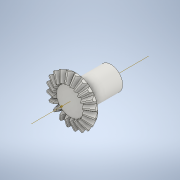
# Autodesk Inventor part: Kegelrad2
Saved by Autodesk Inventor 2021 (Build 250183000, 183)
## iProperties
CustomPartVersion: 1
Created: 2021-01-23
Part Number: Kegelrad2
Material: Steel, Mild
Document SubType Name: Blech
Designer: LETPJG
Categories: <?xml version="1.0" encoding="UTF-16"?> <MemberInstance><Categories><FamilyTemplate><FamilyTemplateParameter ValueType="xs:double" Id="1" ObjectReferenceKey="da_z" ObjectType="kUserParameterObject"/><FamilyTemplateParameter ValueType="xs:double" Id="2" ObjectReferenceKey="da_b" ObjectType="kUserParameterObject"/><FamilyTemplateParameter ValueType="xs:double" Id="3" ObjectReferenceKey="da_beta" ObjectType="kUserParameterObject"/><FamilyTemplateParameter ValueType="xs:double" Id="4" ObjectReferenceKey="da_dae" ObjectType="kUserParameterObject"/><FamilyTemplateParameter ValueType="xs:double" Id="5" ObjectReferenceKey="da_ve" ObjectType="kUserParameterObject"/><FamilyTemplateParameter ValueType="xs:double" Id="6" ObjectReferenceKey="da_omega" ObjectType="kUserParameterObject"/><FamilyTemplateParameter ValueType="xs:string" Id="7" ObjectReferenceKey="EAIAABAAAAAAHwAAAAAAAIAAAAAAAAAA" ObjectType="83914240" SubObjectId="SurfaceGeometry"/></FamilyTemplate><ParamToTemplateMap><ParamToTemplate CategoryParameter="//CategoryParameter[@InternalName='046C89C9-8512-4d59-83FE-43B91F4F132A']" TemplateParameter="1"/><ParamToTemplate CategoryParameter="//CategoryParameter[@InternalName='2552DF32-E462-4b46-AEBF-C6C7768E72AC']" TemplateParameter="2"/><ParamToTemplate CategoryParameter="//CategoryParameter[@InternalName='C9EE641D-15FC-4fae-A226-E94C4372FDD7']" TemplateParameter="3"/><ParamToTemplate><ParamToTemplate CategoryParameter="//CategoryParameter[@InternalName='00B6519A-459B-49c7-AD84-2E56D39A5744']" ConstantValue="-0.000000"/></ParamToTemplate><ParamToTemplate><ParamToTemplate CategoryParameter="//CategoryParameter[@InternalName='04B31F0E-C7A6-4894-AA32-9629BEFACF47']" ConstantValue="1.000000"/></ParamToTemplate><ParamToTemplate><ParamToTemplate CategoryParameter="//CategoryParameter[@InternalName='43CBEC2E-7847-49e7-A936-2F7889FCB2D9']" ConstantValue="0.200000"/></ParamToTemplate><ParamToTemplate><ParamToTemplate CategoryParameter="//CategoryParameter[@InternalName='B1EFC894-105D-4ebd-86BF-FA20ED196853']" ConstantValue="0.300000"/></ParamToTemplate><ParamToTemplate><ParamToTemplate CategoryParameter="//CategoryParameter[@InternalName='51175063-3D10-4879-93E8-6246FE8B403D']" ConstantValue="2060000000.000000"/></ParamToTemplate><ParamToTemplate><ParamToTemplate CategoryParameter="//CategoryParameter[@InternalName='A3A52E27-4454-46a9-B0BD-C932399B70AF']" ConstantValue="0.300000"/></ParamToTemplate><ParamToTemplate CategoryParameter="//CategoryParameter[@InternalName='2A200944-5A8C-41ca-B96E-8520D2E510F1']" TemplateParameter="4"/><ParamToTemplate><ParamToTemplate CategoryParameter="//CategoryParameter[@InternalName='1A637F62-92C8-44bc-B81F-10802510B579']" ConstantValue="1.285835"/></ParamToTemplate><ParamToTemplate CategoryParameter="//CategoryParameter[@InternalName='B52DD4BE-6863-48fb-BF58-89EF6F9EC65C']" TemplateParameter="5"/><ParamToTemplate><ParamToTemplate CategoryParameter="//CategoryParameter[@InternalName='3956BFF2-84D2-457d-93C2-9B0613DEBA67']" ConstantValue="0.252655"/></ParamToTemplate><ParamToTemplate CategoryParameter="//CategoryParameter[@InternalName='739CFA02-461B-4bf8-8049-181FCAD8B28F']" TemplateParameter="6"/><ParamToTemplate><ParamToTemplate CategoryParameter="//CategoryParameter[@InternalName='A27E999F-E2CE-4481-8A2A-EBF499C4C3C5']" ConstantValue="-0.000000"/></ParamToTemplate><ParamToTemplate><ParamToTemplate CategoryParameter="//CategoryParameter[@InternalName='9E1B4470-B2D3-4ff1-B813-535BB4CDF51A']" ConstantValue="3520000.000000"/></ParamToTemplate><ParamToTemplate><ParamToTemplate CategoryParameter="//CategoryParameter[@InternalName='F8452263-BFF6-458c-9FB1-07C4B99E95CD']" ConstantValue="11400000.000000"/></ParamToTemplate><ParamToTemplate><ParamToTemplate CategoryParameter="//CategoryParameter[@InternalName='3E3BB259-FD49-497f-8171-6EBC954A3479']" ConstantValue="2.000000"/></ParamToTemplate><ParamToTemplate CategoryParameter="//CategoryParameter[@InternalName='27C3BAF2-7550-4e4b-AE2C-0DB134B7D9B7']" TemplateParameter="7"/></ParamToTemplateMap><Category DisplayName="Gear" InternalName="DC85795E-93AB-48d5-8EEE-5A27447B64BD" Mnemonic="Gear"><CategoryParameter DisplayName="z" InternalName="046C89C9-8512-4d59-83FE-43B91F4F132A" Mnemonic="z"/><CategoryParameter DisplayName="b" InternalName="2552DF32-E462-4b46-AEBF-C6C7768E72AC" Mnemonic="b"/><CategoryParameter DisplayName="||b|" InternalName="C9EE641D-15FC-4fae-A226-E94C4372FDD7" Mnemonic="beta"/><CategoryParameter DisplayName="x" InternalName="00B6519A-459B-49c7-AD84-2E56D39A5744" Mnemonic="x"/><CategoryParameter DisplayName="a*" InternalName="04B31F0E-C7A6-4894-AA32-9629BEFACF47" Mnemonic="a"/><CategoryParameter DisplayName="c*" InternalName="43CBEC2E-7847-49e7-A936-2F7889FCB2D9" Mnemonic="c"/><CategoryParameter DisplayName="r|.f|*" InternalName="B1EFC894-105D-4ebd-86BF-FA20ED196853" Mnemonic="rf"/><CategoryParameter DisplayName="E" InternalName="51175063-3D10-4879-93E8-6246FE8B403D" Mnemonic="E"/><CategoryParameter DisplayName="||m|" InternalName="A3A52E27-4454-46a9-B0BD-C932399B70AF" Mnemonic="mi"/><Category DisplayName="BevelGear" InternalName="0C98F69A-0C2B-4791-B2FE-7691BB227E77" Mnemonic="BevelGear"><CategoryParameter DisplayName="d|.ae|" InternalName="2A200944-5A8C-41ca-B96E-8520D2E510F1" Mnemonic="dae"/><CategoryParameter DisplayName="d|.ai|" InternalName="1A637F62-92C8-44bc-B81F-10802510B579" Mnemonic="dai"/><CategoryParameter DisplayName="A|.e|" InternalName="B52DD4BE-6863-48fb-BF58-89EF6F9EC65C" Mnemonic="ve"/><CategoryParameter DisplayName="A|.i|" InternalName="3956BFF2-84D2-457d-93C2-9B0613DEBA67" Mnemonic="vi"/><CategoryParameter DisplayName="||S|" InternalName="739CFA02-461B-4bf8-8049-181FCAD8B28F" Mnemonic="omega"/><CategoryParameter DisplayName="x|.t|" InternalName="A27E999F-E2CE-4481-8A2A-EBF499C4C3C5" Mnemonic="xt"/><CategoryParameter DisplayName="||s||.Flim|" InternalName="9E1B4470-B2D3-4ff1-B813-535BB4CDF51A" Mnemonic="sFlim"/><CategoryParameter DisplayName="||s||.Hlim|" InternalName="F8452263-BFF6-458c-9FB1-07C4B99E95CD" Mnemonic="sHlim"/><CategoryParameter DisplayName="Typ" InternalName="3E3BB259-FD49-497f-8171-6EBC954A3479" Mnemonic="type"/><CategoryParameter DisplayName="PitchDiameter" InternalName="27C3BAF2-7550-4e4b-AE2C-0DB134B7D9B7" Mnemonic="IDS_PITCHDIAM"/></Category></Category></Categories></MemberInstance>
Mass: 60.9118 g
Surface Area: 34.3074 cm^2
Volume: 7.7496 cm^3
Density: 7.86 g/cm^3
Appearance: Steel
Sheet Metal Rule: Standard
Author: LETPJG
Autodesk Inventor part; units mm, degrees
ref_plane "Netzebene2" through (0, 0, 0) normal (0.9876883, 0.1564345, 0) x (0, 0, 1)
sketch "Skizze des Zahnradkörpers" plane through (0, 0, 0) normal (1, 0, 0) x (0, 1, 0)
  line L0 (0, 0) -> (9.463344, -6.073313) construction
  line L1 (9.463344, -6.073313) -> (10.447214, -4.105573)
  line L2 (10.447214, -4.105573) -> (0, 0) construction
  line L3 (10, -5) -> (0, 0) construction
  line L4 (5.823707, -3.737494) -> (6.429177, -2.526554)
  line L5 (9.463344, -6.073313) -> (5.823707, -3.737494)
  line L6 (10.447214, -4.105573) -> (6.429177, -2.526554)
  line L7 (0, -39.386751) -> (0, 6.564458)
  line L8 (0, -5) -> (10.447214, -5) construction
  dimension "d0" = 20
  dimension "d1" = 18.92669
  dimension "d2" = 20.89443
  dimension "d3" = 4.3
  dimension "d4" = 4.10557
  constraints: 16 end point, 4 point on line, 3 perpendicular, 2 collinear, 1 horizontal alignment, 1 vertical alignment
  measures "d0" diameter of L3.start L7
  measures "d1" diameter of L0.end L7
  measures "d2" diameter of L1.end L7
  measures "d3" distance between parallel lines of L1 L4
  measures "d4" vertical distance of L1.end L0.start
revolve "Zahnradkörper" add sketch "Skizze des Zahnradkörpers" angle 360 about axis through (0, 0, 0) along (0, 0, 1)
ref_plane "Zahnebene" through (0, 10, -5) normal (0, -0.8944272, 0.4472136) x (1, 0, 0)
sketch "Startskizze" plane through (0, 10, -5) normal (0, -0.8944272, 0.4472136) x (1, 0, 0)
  line L0 (0, -23.505131) -> (0, 10.644758)
  arc A0 (-0.366347, -1.464) -> (-1.669997, 1.601878) centre (-8.211235, -2.989641) ccw
  arc A1 (1.669997, 1.601878) -> (0.366347, -1.464) centre (8.211235, -2.989641) ccw
  line L1 (-0.366347, -1.464) -> (0.366347, -1.464)
  arc A2 (1.669997, 1.601878) -> (-1.669997, 1.601878) centre (0, -22.36068) ccw
  dimension "d7" = 7.99186
  dimension "d8" = 8.21124
  dimension "d9" = 19.37104
  dimension "d57" = 24.02068
  dimension "d58" = 20.89668
  constraints: 6 point on circle, 3 centre point, 3 symmetric about line, 2 end point, 1 coincident, 1 perpendicular, 1 other
  measures "d7" radius of A0
  measures "d8" horizontal distance of point (0, -22.361) A0.centre
  measures "d9" vertical distance of point (0, -22.361) A0.centre
  measures "d57" radius of A2
  measures "d58" distance from line of A2.centre L1
ref_plane "Endebene" through (0, 6.055576, -3.027788) normal (0, -0.8944272, 0.4472136) x (1, 0, 0)
sketch "Endskizze" plane through (0, 6.055576, -3.027788) normal (0, -0.8944272, 0.4472136) x (1, 0, 0)
  line L0 (0, -15.35404) -> (0, 6.953444)
  arc A0 (-0.221844, -0.886536) -> (-1.011279, 0.970029) centre (-4.972376, -1.8104) ccw
  arc A1 (1.011279, 0.970029) -> (0.221844, -0.886536) centre (4.972376, -1.8104) ccw
  line L1 (-0.221844, -0.886536) -> (0.221844, -0.886536)
  arc A2 (1.011279, 0.970029) -> (-1.011279, 0.970029) centre (0, -13.54068) ccw
  dimension "d12" = 4.83953
  dimension "d15" = 4.97238
  dimension "d16" = 11.73028
  dimension "d59" = 14.54591
  dimension "d60" = 12.65414
  constraints: 6 point on circle, 3 centre point, 3 symmetric about line, 2 end point, 1 coincident, 1 other
  measures "d12" radius of A0
  measures "d15" horizontal distance of A0.centre point (0, -13.541)
  measures "d16" vertical distance of A0.centre point (0, -13.541)
  measures "d59" radius of A2
  measures "d60" distance from line of A2.centre L1
loft "Loft" cut profiles "Startskizze", "Endskizze"
pattern_circular "Circular Pattern" count 20 over 360 about axis through (0, 0, 0) along (0, 0, 1) of "Loft"
sketch3d "3D-Skizze rechts"
ref_plane "Endebene rechts" through (-1.195497, 5.936395, -3.027788) normal (0.1765786, -0.8768238, 0.4472136) x (0.9803188, 0.1974209, 0)
sketch "Endskizze rechts" plane through (-1.195497, 5.936395, -3.027788) normal (0.1765786, -0.8768238, 0.4472136) x (0.9803188, 0.1974209, 0)
  arc A0 (-0.221844, -0.886536) -> (-1.011279, 0.970029) centre (-4.972376, -1.8104) ccw
  line L0 (0, -18.59884) -> (0, 8.824815)
  arc A1 (1.011279, 0.970029) -> (0.221844, -0.886536) centre (4.972376, -1.8104) ccw
  line L1 (-0.221844, -0.886536) -> (0.221844, -0.886536)
  arc A2 (1.011279, 0.970029) -> (-1.011279, 0.970029) centre (0, -13.54068) ccw
  dimension "d70" = 4.97238
  dimension "d71" = 11.73028
  dimension "d72" = 4.83953
  dimension "d73" = 12.65414
  dimension "d74" = 14.54591
  constraints: 6 point on circle, 3 centre point, 3 symmetric about line, 2 end point, 1 coincident, 1 perpendicular, 1 other
  measures "d70" horizontal distance of A2.centre A0.centre
  measures "d71" vertical distance of point (0, -13.541) A0.centre
  measures "d72" radius of A0
  measures "d73" distance from line of point (0, -13.541) L1
  measures "d74" radius of A2
feature "Erhebung rechts" [suppressed]
pattern_circular "Runde Anordnung rechts" [suppressed]
sketch3d "3D-Skizze links"
ref_plane "Endebene links" through (1.238266, 5.936395, -3.054356) normal (-0.1823679, -0.8742937, 0.449836) x (0.9789304, -0.204194, 0)
sketch "Endskizze links" plane through (1.238266, 5.936395, -3.054356) normal (-0.1823679, -0.8742937, 0.449836) x (0.9789304, -0.204194, 0)
  line L0 (0, -29.014384) -> (0, 11.991661)
  arc A0 (-0.221844, -0.866613) -> (-1.011279, 0.989952) centre (-4.972376, -1.790477) ccw
  arc A1 (1.011279, 0.989952) -> (0.221844, -0.866613) centre (4.972376, -1.790477) ccw
  line L1 (-0.221844, -0.866613) -> (0.221844, -0.866613)
  ellipse E0 centre (0, -2.256494) end of major axis (6.429177, -2.256494) minor radius 2.892075
  arc A2 (1.011279, 0.989952) -> (-1.011279, 0.989952) centre (0, -13.520757) ccw
  dimension "d56" = 2.89207
  dimension "d30" = 4.83953
  dimension "d31" = 4.97238
  dimension "d32" = 11.73028
  dimension "d61" = 14.54591
  dimension "d62" = 12.65414
  constraints: 6 point on circle, 3 centre point, 3 symmetric about line, 2 end point, 1 coincident, 2 other
  measures "d30" radius of A0
  measures "d31" horizontal distance of point (0, -13.521) A0.centre
  measures "d32" vertical distance of A0.centre point (0, -13.521)
  measures "d61" radius of A2
  measures "d62" distance from line of point (0, -13.521) L1
feature "Erhebung links" [suppressed]
pattern_circular "Runde Anordnung links" [suppressed]
sketch "Körperskizze" plane through (0, 0, 0) normal (1, 0, 0) x (0, 1, 0)
  line L0 (0, -35.037536) -> (0, -19.530831)
  line L1 (9.463344, -6.073313) -> (5.823707, -3.737494)
  line L2 (5.823707, -3.737494) -> (0, -3.737494)
  line L3 (9.463344, -6.073313) -> (0, -6.073313)
  constraints: 4 end point, 2 perpendicular, 2 point on line
sketch "Körperskizze outline for Festkörper" plane through (0, 0, 0) normal (1, 0, 0) x (0, 1, 0)
  line L0 (0, -6.073313) -> (9.463344, -6.073313)
  line L1 (0, -3.737494) -> (0, -6.073313)
  line L2 (5.823707, -3.737494) -> (0, -3.737494)
  line L3 (9.463344, -6.073313) -> (5.823707, -3.737494)
revolve "Festkörper" add sketch "Körperskizze outline for Festkörper" angle 360 about axis through (0, 0, 0) along (0, 0, 1)
sketch "Sketch6" plane through (0, 0, 0) normal (1, 0, 0) x (0, 1, 0)
  line L0 (10, -5) -> (0, 0)
  line L1 (0, -37.799919) -> (0, 6.299986)
surface revolve "Flankendurchmesser" sketch "Sketch6" angle 360 about axis through (0, 0, 0) along (0, 0, 1) shown no curves L0
sketch "Skizze8" plane through (0, 0, -6.073313) normal (0, 0, -1) x (-1, 0, 0)
  circle A0 centre (0, 0) radius 5
  dimension "d94" = 10
  constraints: 1 centre point, 1 coincident
  measures "d94" diameter of A0
extrude "Extrusion1" add sketch "Skizze8" along normal blind 15
equation "\"d0\" = da_de"
equation "\"d1\" = da_dfe"
equation "\"d2\" = da_dae"
equation "\"d3\" = da_b"
equation "\"d4\" = da_ve"
equation "\"d7\" = fd_rr"
equation "\"d8\" = fd_x"
equation "\"d9\" = fd_y"
equation "\"d57\" = 0.5 * fd_dva + 0.3 * da_he"
equation "\"d58\" = 0.5 * fd_dva - 1.12 * da_he"
equation "\"da_teethtype\" = 0"
equation "\"da_b\" = 4.3"
equation "\"da_de\" = 20"
equation "\"da_dae\" = 20.89443"
equation "\"da_dfe\" = 18.92669"
equation "\"da_le\" = 11.18034"
equation "\"da_omega\" = 90deg"
equation "\"da_beta\" = 0"
equation "\"da_delta\" = 63.434949deg"
equation "\"da_alpha\" = 20deg"
equation "\"da_he\" = 2.2"
equation "\"da_ve\" = 4.10557"
equation "\"da_zv\" = 44.72136"
equation "\"fd_loft\" = da_b + 0.05 * da_he"
equation "\"fd_x\" = fd_x1 + fd_x2"
equation "\"fd_y\" = fd_y1 - fd_y2"
equation "\"fd_dd\" = fd_dva - 0.8 * da_he"
equation "\"da_dvw\" = 44.72136"
equation "\"d11\" = fd_loft"
equation "\"da_dm\" = 16.15396"
equation "\"da_x\" = 0"
equation "\"da_m\" = 1"
equation "\"d50\" = da_omega"
equation "\"Biegeradius\" = Stärke"
equation "\"BreiteBiegungsfreistellung\" = Stärke"
equation "\"TiefeBiegungsfreistellung\" = 0.5 * Stärke"
equation "\"GrößeEckenfreistellung\" = 4 * Stärke"
equation "\"MinimalRest\" = 2 * Stärke"
equation "\"Übergangsradius\" = Biegeradius"
equation "\"JacobiRadiusGröße\" = Stärke"
equation "\"Abstandsgröße\" = Stärke"
equation "\"fd_rr\" = 7.991862"
equation "\"fd_dva\" = 46.72136"
equation "\"fd_x1\" = 0.793958"
equation "\"fd_x2\" = 7.417277"
equation "\"fd_y1\" = 22.34658"
equation "\"fd_y2\" = 2.975542"
equation "\"Stärke\" = 0.5"
body "Solid1"
body "Srf1"
